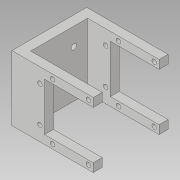
# Autodesk Inventor part: connection_hand
Saved by Autodesk Inventor 2017 (Build 210142000, 142)
## iProperties
Part Number: connection_hand
Material: Aluminium 6061
Document SubType Name: Modeling
Designer: Max
Density: 2.7 g/cm^3
Appearance: Vorgabe
Mass: 33.2037 g
Surface Area: 85.4905 cm^2
Volume: 12.2977 cm^3
Author: Max
Autodesk Inventor part; units mm, degrees
ref_plane "YZ Plane" through (0, 0, 0) normal (1, 0, 0) x (0, 1, 0)
ref_plane "XZ Plane" through (0, 0, 0) normal (0, 1, 0) x (-1, 0, 0)
ref_plane "XY Plane" through (0, 0, 0) normal (0, 0, 1) x (1, 0, 0)
sketch "Skizze1" plane through (0, 0, 0) normal (1, 0, 0) x (0, 1, 0)
  line L0 (-23, 20) -> (23, 20)
  line L1 (23, 20) -> (23, -20)
  line L2 (23, -20) -> (-23, -20)
  line L3 (-23, -20) -> (-23, 20)
  line L4 (-23, 20) -> (23, -20) construction
  line L5 (23, 20) -> (-23, -20) construction
  point P0 (0, 0)
  dimension "d0" = 46
  dimension "d1" = 40
  constraints: 12 end point, 2 midpoint, 2 parallel, 1 horizontal, 1 perpendicular
  measures "d0" distance of L1.end L2.end
  measures "d1" distance of L0.end L1.end
extrude "Extrusion1" add sketch "Skizze1" along normal blind 50
sketch "Skizze2" plane through (0, -23, 20) normal (0, 0, 1) x (1, 0, 0)
  line L0 (0, 0) -> (0, 46) projected
  line L1 (0, 0) -> (50, 0) projected
  line L2 (50, 46) -> (50, 0) projected
  line L3 (0, 46) -> (50, 46) projected
  line L4 (50, 46) -> (50, 0) projected
  line L5 (50, 40.5) -> (6, 40.5)
  line L6 (6, 40.5) -> (6, 5.5)
  line L7 (6, 5.5) -> (50, 5.5)
  line L8 (50, 5.5) -> (50, 40.5)
  point P0 (0, 23)
  dimension "d4" = 5.5
  dimension "d5" = 5.5
  dimension "d6" = 6
  constraints: 8 end point, 2 parallel, 1 horizontal, 1 perpendicular, 1 point on line
  measures "d4" distance between parallel lines of L5 L3
  measures "d5" distance between parallel lines of L1 L7
  measures "d6" distance between parallel lines of L0 L6
extrude "Extrusion2" cut sketch "Skizze2" against normal through all contours L7 L6 L5 L2
sketch "Skizze3" plane through (0, -23, -20) normal (0, -1, 0) x (1, 0, 0)
  line L0 (0, 0) -> (0, 40) projected
  line L1 (0, 0) -> (50, 0) projected
  line L2 (50, 40) -> (50, 0) projected
  line L3 (0, 40) -> (50, 40) projected
  line L4 (0, 20) -> (44.7617, 20) construction
  line L5 (20, 34.75) -> (50, 34.75)
  line L6 (50, 34.75) -> (50, 5.25)
  line L7 (50, 5.25) -> (20, 5.25)
  line L8 (20, 5.25) -> (20, 34.75)
  line L9 (20, 34.75) -> (50, 5.25) construction
  line L10 (50, 34.75) -> (20, 5.25) construction
  point P0 (35, 20)
  dimension "d9" = 29.5
  dimension "d10" = 30
  constraints: 14 end point, 2 horizontal, 2 midpoint, 2 parallel, 2 point on line, 1 perpendicular
  measures "d9" distance of L7.end L5.start
  measures "d10" distance of L6.end L7.end
extrude "Extrusion3" cut sketch "Skizze3" against normal through all contours L7 L8 L5 L2
sketch "Skizze4" plane through (0, -23, -20) normal (0, -1, 0) x (1, 0, 0)
  line L0 (50, 5.25) -> (20, 5.25) projected
  line L1 (20, 5.25) -> (20, 34.75) projected
  line L2 (20, 34.75) -> (50, 34.75) projected
  line L3 (50, 40) -> (50, 34.75) projected
  line L4 (0, 40) -> (50, 40) projected
  line L5 (0, 0) -> (0, 40) projected
  line L6 (0, 0) -> (50, 0) projected
  line L7 (50, 5.25) -> (50, 0) projected
  line L8 (0, 20) -> (84.4351, 20) construction
  point P0 (25, 37.3)
  point P1 (25, 2.7)
  point P2 (17.2, 31)
  point P3 (17.2, 9)
  point P4 (47, 37.3)
  point P5 (47, 2.7)
  dimension "d13" = 5
  dimension "d14" = 5
  dimension "d15" = 34.6
  dimension "d16" = 17.3
  dimension "d17" = 22
  dimension "d18" = 11
  dimension "d19" = 2.8
  dimension "d20" = 2.8
  dimension "d47" = 17.3
  dimension "d48" = 17.3
  dimension "d49" = 22
  dimension "d50" = 22
  constraints: 2 end point, 1 horizontal
  measures "d13" distance from line of point (25, 2.7) L1
  measures "d14" distance from line of L1 point (25, 37.3)
  measures "d15" distance of point (25, 2.7) point (25, 37.3)
  measures "d16" distance from line of L8 point (25, 37.3)
  measures "d17" distance of point (17.2, 9) point (17.2, 31)
  measures "d18" distance from line of L8 point (17.2, 31)
  measures "d19" distance from line of L1 point (17.2, 31)
  measures "d20" distance from line of L1 point (17.2, 9)
  measures "d47" distance from line of point (47, 37.3) L8
  measures "d48" distance from line of L8 point (47, 2.7)
  measures "d49" distance of point (47, 37.3) point (25, 37.3)
  measures "d50" distance of point (47, 2.7) point (25, 2.7)
hole "Bohrung1" at (25, -23, 17.3) at (25, -23, -17.3) at (17.2, -23, 11) at (17.2, -23, -11) at (47, -23, 17.3) at (47, -23, -17.3) direction (0, 1, 0) diameter 2.9 end through all clearance for "Inbusschraube ISO 4762" size "M2.5" standard "ISO"
sketch "Skizze7" plane through (6, -17.5, 20) normal (1, 0, 0) x (0, 0, -1)
  line L0 (29, 8.5) -> (11, 8.5)
  line L1 (11, 8.5) -> (11, 26.5)
  line L2 (11, 26.5) -> (29, 26.5)
  line L3 (29, 26.5) -> (29, 8.5)
  line L4 (29, 8.5) -> (11, 26.5) construction
  line L5 (11, 8.5) -> (29, 26.5) construction
  point P0 (20, 17.5)
  dimension "d52" = 18
  dimension "d53" = 18
  constraints: 12 end point, 2 midpoint, 2 parallel, 1 horizontal, 1 perpendicular
  measures "d52" distance of L1.end L2.end
  measures "d53" distance of L0.end L1.end
hole "Bohrung3" at (6, -9, 9) at (6, 9, 9) at (6, 9, -9) at (6, -9, -9) direction (-1, 0, 0) diameter 3.4 end through all clearance for "Inbusschraube ISO 4762" size "M3" standard "ISO"
equation "\"d5\" = d4"
equation "\"d13\" = d14"
equation "\"d16\" = 0.5 * d15"
equation "\"d18\" = 0.5 * d17"
equation "\"d20\" = d19"
equation "\"d47\" = d16"
equation "\"d48\" = d16"
equation "\"d50\" = d49"
equation "\"d53\" = d52"
